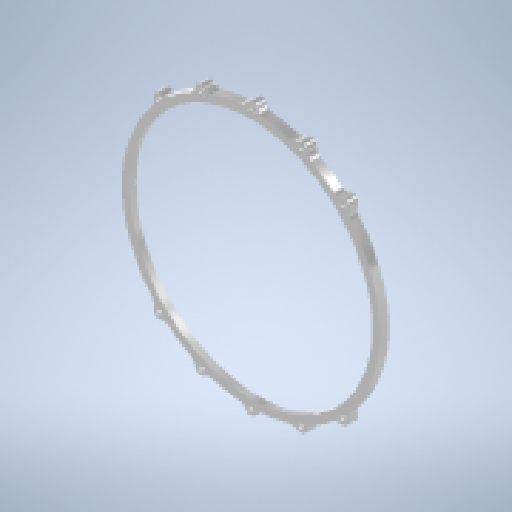
# Autodesk Inventor part: 出力ベアリング抑え
Saved by Autodesk Inventor 2024 (Build 280153000, 153)
## iProperties
Created: 2023-05-29
Part Number: 出力ベアリング抑え
Material: アルミニウム 6061
Document SubType Name: Modeling
Designer: yuta2
Density: 2.7 g/cm^3
Appearance: アルミニウム - フラット
Author: yuta2
Autodesk Inventor part; units mm, degrees
ref_plane "YZ Plane" through (0, 0, 0) normal (1, 0, 0) x (0, 1, 0)
ref_plane "XZ Plane" through (0, 0, 0) normal (0, 1, 0) x (-1, 0, 0)
ref_plane "XY Plane" through (0, 0, 0) normal (0, 0, 1) x (1, 0, 0)
sketch "スケッチ1" plane through (0, 0, 0) normal (0, 0, 1) x (1, 0, 0)
  circle A0 centre (0, 0) radius 61
  circle A1 centre (0, 0) radius 65
  dimension "d0" = 122
  dimension "d1" = 130
  constraints: 2 centre point, 2 coincident
  measures "d0" diameter of A0
  measures "d1" diameter of A1
extrude "押し出し1" add sketch "スケッチ1" along normal blind 2.5
sketch "スケッチ2" plane through (0, 0, 0) normal (0, 0, -1) x (-1, 0, 0)
  circle A0 centre (0, 0) radius 65 projected
  circle A1 centre (0, 0) radius 61 projected
  circle A2 centre (0, 0) radius 62.5
  dimension "d4" = 125
  constraints: 1 centre point, 1 coincident
  measures "d4" diameter of A2
extrude "押し出し2" add sketch "スケッチ2" along normal blind 2.5 contours A0
sketch "スケッチ3" plane through (0, 0, 2.5) normal (0, 0, 1) x (1, 0, 0)
  circle A0 centre (0, 0) radius 65 projected
  circle A1 centre (0, 0) radius 62.5 projected
  circle A2 centre (0, 65.5) radius 3
  point P0 (2.946, 64.9332)
  point P1 (-2.946, 64.9332)
  dimension "d7" = 6
  constraints: 1 centre point, 1 tangent, 1 vertical alignment
  measures "d7" diameter of A2
extrude "押し出し3" add sketch "スケッチ3" against normal blind 5 contours A0 A2 picked at (-0.0949, 66.1572)
fillet "フィレット1" radius 5 4 edges at (2.946, 64.9332, 1.25) (2.946, 64.9332, -1.25) (-2.946, 64.9332, 1.25) (-2.946, 64.9332, -1.25)
pattern_circular "円形状パターン1" count 16 over 360 about axis through (0, 0, 0) along (0, 0, 1) of "押し出し3", "フィレット1"
sketch "スケッチ4" plane through (0, 0, 2.5) normal (0, 0, 1) x (1, 0, 0)
  arc A0 (-6.3418, 64.6899) -> (-18.8967, 62.1926) centre (0, 0) ccw projected
  arc A1 (-23.2974, 62.9375) -> (-18.8967, 62.1926) centre (-20.3503, 66.9766) ccw projected
  arc A2 (-23.2974, 62.9375) -> (-28.0298, 60.9774) centre (-25.0658, 60.5141) ccw projected
  arc A3 (-30.6148, 57.3388) -> (-28.0298, 60.9774) centre (-32.9698, 61.7494) ccw projected
  arc A4 (-30.6148, 57.3388) -> (-41.2583, 50.227) centre (0, 0) ccw projected
  arc A5 (-45.6092, 49.2312) -> (-41.2583, 50.227) centre (-44.432, 54.0906) ccw projected
  arc A6 (-45.6092, 49.2312) -> (-49.2312, 45.6092) centre (-46.3155, 46.3155) ccw projected
  arc A7 (-50.227, 41.2583) -> (-49.2312, 45.6092) centre (-54.0906, 44.432) ccw projected
  arc A8 (-50.227, 41.2583) -> (-57.3388, 30.6148) centre (0, 0) ccw projected
  arc A9 (-60.9774, 28.0298) -> (-57.3388, 30.6148) centre (-61.7494, 32.9698) ccw projected
  arc A10 (-60.9774, 28.0298) -> (-62.9375, 23.2974) centre (-60.5141, 25.0658) ccw projected
  arc A11 (-62.1926, 18.8967) -> (-62.9375, 23.2974) centre (-66.9766, 20.3503) ccw projected
  arc A12 (-62.1926, 18.8967) -> (-64.6899, 6.3418) centre (0, 0) ccw projected
  arc A13 (-67.0623, 2.5611) -> (-64.6899, 6.3418) centre (-69.666, 6.8297) ccw projected
  arc A14 (-67.0623, 2.5611) -> (-67.0623, -2.5611) centre (-65.5, 0) ccw projected
  arc A15 (-64.6899, -6.3418) -> (-67.0623, -2.5611) centre (-69.666, -6.8297) ccw projected
  arc A16 (-64.6899, -6.3418) -> (-62.1926, -18.8967) centre (0, 0) ccw projected
  arc A17 (-62.9375, -23.2974) -> (-62.1926, -18.8967) centre (-66.9766, -20.3503) ccw projected
  arc A18 (-62.9375, -23.2974) -> (-60.9774, -28.0298) centre (-60.5141, -25.0658) ccw projected
  arc A19 (-57.3388, -30.6148) -> (-60.9774, -28.0298) centre (-61.7494, -32.9698) ccw projected
  arc A20 (-57.3388, -30.6148) -> (-50.227, -41.2583) centre (0, 0) ccw projected
  arc A21 (-49.2312, -45.6092) -> (-50.227, -41.2583) centre (-54.0906, -44.432) ccw projected
  arc A22 (-49.2312, -45.6092) -> (-45.6092, -49.2312) centre (-46.3155, -46.3155) ccw projected
  arc A23 (-41.2583, -50.227) -> (-45.6092, -49.2312) centre (-44.432, -54.0906) ccw projected
  arc A24 (-41.2583, -50.227) -> (-30.6148, -57.3388) centre (0, 0) ccw projected
  arc A25 (-28.0298, -60.9774) -> (-30.6148, -57.3388) centre (-32.9698, -61.7494) ccw projected
  arc A26 (-28.0298, -60.9774) -> (-23.2974, -62.9375) centre (-25.0658, -60.5141) ccw projected
  arc A27 (-18.8967, -62.1926) -> (-23.2974, -62.9375) centre (-20.3503, -66.9766) ccw projected
  arc A28 (-18.8967, -62.1926) -> (-6.3418, -64.6899) centre (0, 0) ccw projected
  arc A29 (-2.5611, -67.0623) -> (-6.3418, -64.6899) centre (-6.8297, -69.666) ccw projected
  arc A30 (-2.5611, -67.0623) -> (2.5611, -67.0623) centre (0, -65.5) ccw projected
  arc A31 (6.3418, -64.6899) -> (2.5611, -67.0623) centre (6.8297, -69.666) ccw projected
  arc A32 (6.3418, -64.6899) -> (18.8967, -62.1926) centre (0, 0) ccw projected
  arc A33 (23.2974, -62.9375) -> (18.8967, -62.1926) centre (20.3503, -66.9766) ccw projected
  arc A34 (23.2974, -62.9375) -> (28.0298, -60.9774) centre (25.0658, -60.5141) ccw projected
  arc A35 (30.6148, -57.3388) -> (28.0298, -60.9774) centre (32.9698, -61.7494) ccw projected
  arc A36 (30.6148, -57.3388) -> (41.2583, -50.227) centre (0, 0) ccw projected
  arc A37 (45.6092, -49.2312) -> (41.2583, -50.227) centre (44.432, -54.0906) ccw projected
  arc A38 (45.6092, -49.2312) -> (49.2312, -45.6092) centre (46.3155, -46.3155) ccw projected
  arc A39 (50.227, -41.2583) -> (49.2312, -45.6092) centre (54.0906, -44.432) ccw projected
  arc A40 (50.227, -41.2583) -> (57.3388, -30.6148) centre (0, 0) ccw projected
  arc A41 (60.9774, -28.0298) -> (57.3388, -30.6148) centre (61.7494, -32.9698) ccw projected
  arc A42 (60.9774, -28.0298) -> (62.9375, -23.2974) centre (60.5141, -25.0658) ccw projected
  arc A43 (62.1926, -18.8967) -> (62.9375, -23.2974) centre (66.9766, -20.3503) ccw projected
  arc A44 (62.1926, -18.8967) -> (64.6899, -6.3418) centre (0, 0) ccw projected
  arc A45 (67.0623, -2.5611) -> (64.6899, -6.3418) centre (69.666, -6.8297) ccw projected
  arc A46 (67.0623, -2.5611) -> (67.0623, 2.5611) centre (65.5, 0) ccw projected
  arc A47 (64.6899, 6.3418) -> (67.0623, 2.5611) centre (69.666, 6.8297) ccw projected
  arc A48 (64.6899, 6.3418) -> (62.1926, 18.8967) centre (0, 0) ccw projected
  arc A49 (62.9375, 23.2974) -> (62.1926, 18.8967) centre (66.9766, 20.3503) ccw projected
  arc A50 (62.9375, 23.2974) -> (60.9774, 28.0298) centre (60.5141, 25.0658) ccw projected
  arc A51 (57.3388, 30.6148) -> (60.9774, 28.0298) centre (61.7494, 32.9698) ccw projected
  arc A52 (57.3388, 30.6148) -> (50.227, 41.2583) centre (0, 0) ccw projected
  arc A53 (49.2312, 45.6092) -> (50.227, 41.2583) centre (54.0906, 44.432) ccw projected
  arc A54 (49.2312, 45.6092) -> (45.6092, 49.2312) centre (46.3155, 46.3155) ccw projected
  arc A55 (41.2583, 50.227) -> (45.6092, 49.2312) centre (44.432, 54.0906) ccw projected
  arc A56 (41.2583, 50.227) -> (30.6148, 57.3388) centre (0, 0) ccw projected
  arc A57 (28.0298, 60.9774) -> (30.6148, 57.3388) centre (32.9698, 61.7494) ccw projected
  arc A58 (28.0298, 60.9774) -> (23.2974, 62.9375) centre (25.0658, 60.5141) ccw projected
  arc A59 (18.8967, 62.1926) -> (23.2974, 62.9375) centre (20.3503, 66.9766) ccw projected
  arc A60 (18.8967, 62.1926) -> (6.3418, 64.6899) centre (0, 0) ccw projected
  arc A61 (2.5611, 67.0623) -> (6.3418, 64.6899) centre (6.8297, 69.666) ccw projected
  arc A62 (2.5611, 67.0623) -> (-2.5611, 67.0623) centre (0, 65.5) ccw projected
  arc A63 (-6.3418, 64.6899) -> (-2.5611, 67.0623) centre (-6.8297, 69.666) ccw projected
  circle A64 centre (0, 0) radius 61 projected
  circle A65 centre (0, 0) radius 65
  point P0 (62.1926, -18.8967)
  point P1 (57.3388, -30.6148)
  point P2 (64.6899, 6.3418)
  point P3 (57.3388, 30.6148)
  point P4 (62.1926, 18.8967)
  point P5 (-57.3388, -30.6148)
  point P6 (-62.1926, -18.8967)
  point P7 (-64.6899, -6.3418)
  point P8 (-64.6899, 6.3418)
  point P9 (-62.1926, 18.8967)
  point P10 (-57.3388, 30.6148)
  constraints: 1 centre point, 1 coincident, 1 concentric
extrude "押し出し4" cut sketch "スケッチ4" against normal through all contours A65 A11 A10 A9 | A51 A50 A49 A65 | A65 A15 A14 A13 | A47 A46 A45 A65 | A65 A19 A18 A17 | A43 A42 A41 A65
sketch "スケッチ5" plane through (0, 0, 2.5) normal (0, 0, 1) x (1, 0, 0)
  arc A0 (-45.6092, 49.2312) -> (-49.2312, 45.6092) centre (-46.3155, 46.3155) ccw projected
  arc A1 (-23.2974, 62.9375) -> (-28.0298, 60.9774) centre (-25.0658, 60.5141) ccw projected
  arc A2 (2.5611, 67.0623) -> (-2.5611, 67.0623) centre (0, 65.5) ccw projected
  arc A3 (28.0298, 60.9774) -> (23.2974, 62.9375) centre (25.0658, 60.5141) ccw projected
  arc A4 (49.2312, 45.6092) -> (45.6092, 49.2312) centre (46.3155, 46.3155) ccw projected
  arc A5 (45.6092, -49.2312) -> (49.2312, -45.6092) centre (46.3155, -46.3155) ccw projected
  arc A6 (23.2974, -62.9375) -> (28.0298, -60.9774) centre (25.0658, -60.5141) ccw projected
  arc A7 (-2.5611, -67.0623) -> (2.5611, -67.0623) centre (0, -65.5) ccw projected
  arc A8 (-28.0298, -60.9774) -> (-23.2974, -62.9375) centre (-25.0658, -60.5141) ccw projected
  arc A9 (-49.2312, -45.6092) -> (-45.6092, -49.2312) centre (-46.3155, -46.3155) ccw projected
  point P0 (0, 0)
  constraints: 10 coincident
hole "穴1" at (-46.3155, 46.3155, 2.5) at (-25.0658, 60.5141, 2.5) at (0, 65.5, 2.5) at (25.0658, 60.5141, 2.5) at (46.3155, 46.3155, 2.5) at (46.3155, -46.3155, 2.5) at (25.0658, -60.5141, 2.5) at (0, -65.5, 2.5) at (-25.0658, -60.5141, 2.5) at (-46.3155, -46.3155, 2.5) direction (0, 0, -1) diameter 3.3 end through all
